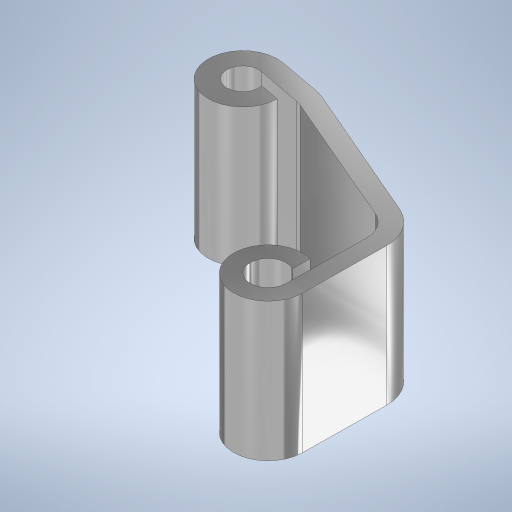
# Autodesk Inventor part: Linkage for half overlay hinge
Saved by Autodesk Inventor 2024 (Build 280153000, 153)
## iProperties
Category: Perkama detale
Created: 2008-03-26
Part Number: Linkage for half overlay hinge
Document SubType Name: Modeling
Designer: G.K.
Material: Steel
Description: Linkage for half overlay hinge
Authority: Design by UAB Čeli APS
Mass: 4.16659 g
Surface Area: 9.6431 cm^2
Volume: 0.530776 cm^3
Density: 7.85 g/cm^3
Appearance: Chrome - Polished
Mase: 0.00416659
Author: Kestas
Autodesk Inventor part; units mm, degrees
ref_plane "YZ Plane" through (0, 0, 0) normal (1, 0, 0) x (0, 1, 0)
ref_plane "XZ Plane" through (0, 0, 0) normal (0, 1, 0) x (-1, 0, 0)
ref_plane "XY Plane" through (0, 0, 0) normal (0, 0, 1) x (1, 0, 0)
sketch "Sketch1" plane through (0, 0, 0) normal (0, 0, 1) x (1, 0, 0)
  arc A0 (6.0128, 43.747) -> (6.9228, 42.8627) centre (5.7994, 42.6169) ccw
  arc A1 (6.2634, 45.0735) -> (8.2994, 42.6027) centre (5.7994, 42.6169) ccw
  arc A2 (19.5106, 33.7857) -> (21.381, 31.3359) centre (18.8812, 31.3663) ccw
  line L0 (6.2634, 45.0735) -> (9.5295, 44.4566)
  line L1 (9.5295, 44.4566) -> (21.4782, 39.3353)
  line L2 (21.4782, 39.3353) -> (21.381, 31.3359)
  line L3 (6.0128, 43.747) -> (9.3605, 43.1146)
  line L4 (9.3605, 43.1146) -> (20.2673, 38.4399)
  line L5 (20.2673, 38.4399) -> (20.1811, 31.3505)
  line L6 (6.9228, 42.8627) -> (8.2994, 42.6027)
  line L7 (19.5106, 33.7857) -> (19.4952, 32.5121)
  arc A3 (19.4952, 32.5121) -> (20.1811, 31.3505) centre (18.8812, 31.3663) ccw
  line L8 (5.7994, 42.6169) -> (18.8812, 31.3663) construction
  arc A4 (6.9392, 42.2416) -> (4.6204, 42.3936) centre (5.7994, 42.6169) ccw
  point P0 (0, 0)
  dimension "d0" = 5
  dimension "d1" = 5
  dimension "d2" = 1.3
  dimension "d5" = 1.35
  dimension "d8" = 8
  dimension "d9" = 0.7
  dimension "d10" = 0.7
  dimension "d12" = 1.2
  dimension "d18" = 2.3
  dimension "d19" = 30
  dimension "d20" = 13
  dimension "d21" = 50
  constraints: 18 end point, 10 point on circle, 5 centre point, 5 parallel, 4 tangent, 2 coincident, 6 other
  measures "d0" diameter of A1
  measures "d1" diameter of A2
  measures "d2" distance between parallel lines of L1 L4
  measures "d5" distance between parallel lines of L3 L0
  measures "d8" distance of L1.end L2.end
  measures "d9" distance between parallel lines of L3 L6
  measures "d10" distance between parallel lines of L5 L7
  measures "d12" distance between parallel lines of L2 L5
  measures "d18" diameter of A0
  measures "d19" angle of L8 L3
  measures "d20" distance of L0.end L1.end
  measures "d21" angle of L8 L5
extrude "Extrusion1" add sketch "Sketch1" along normal mid plane 10 contours A0 L6 A1 L0 L1 L2 A2 L7 A3 L5 L4 L3
fillet "Fillet1" radius 2 2 edges at (20.2673, 38.4399, 0) (9.3605, 43.1146, 0)
fillet "Fillet1" radius 3 2 edges at (9.5295, 44.4566, 0) (21.4782, 39.3353, 0)
body "Solid1"
